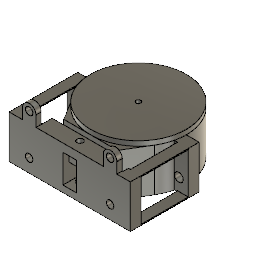
dropgen_assembly (Autodesk Fusion 360 archive; units mm, degrees)
design "drop_gen_reservoir"
Autodesk Fusion 360 part; units mm, degrees
sketch "Sketch1" plane through (0, 0, 0) normal (0, 1, 0) x (1, 0, 0) in component "reservoir assembly"
  line L0 (-25, 0) -> (25, 0)
  line L1 (25, 0) -> (25, 16)
  line L2 (25, 16) -> (-25, 16)
  line L3 (-25, 16) -> (-25, 0)
  line L4 (25, 0) -> (28.5, 0)
  line L5 (28.5, 0) -> (28.5, 19)
  line L6 (28.5, 19) -> (32, 19)
  line L7 (32, 19) -> (32, -5)
  line L8 (32, -5) -> (35.5, -5)
  line L9 (35.5, -5) -> (35.5, 27)
  line L10 (35.5, 27) -> (0, 27)
  line L11 (0, 0) -> (0, 27) construction
  line L12 (0, 16) -> (0, 27)
  line L13 (0, -8.5) -> (35.5, -8.5)
  line L14 (35.5, -8.5) -> (35.5, -5)
  line L15 (35.5, -5) -> (31.85, -5)
  line L16 (31.85, -5) -> (31.85, -3.5)
  line L17 (31.85, -3.5) -> (0, -3.5)
  line L18 (0, -3.5) -> (0, -8.5)
  line L19 (0, 16) -> (25, 8)
  line L20 (25, 0) -> (25, 8)
  dimension "d1" = 50
  dimension "d2" = 16
  dimension "d3" = 3.5
  dimension "d4" = 3.5
  dimension "d5" = 3.5
  dimension "d6" = 5
  dimension "d10" = 1.5
  dimension "d11" = 0.15
  dimension "d13" = 3.5
  dimension "d18" = 8
  dimension "d24" = 3
  dimension "d25" = 8
  constraint horizontal L0
  constraint vertical L1
  constraint horizontal L2
  constraint vertical L3
  constraint midpoint L11.start L0
  constraint perpendicular L1 L4
  constraint perpendicular L4 L5
  constraint perpendicular L5 L6
  constraint perpendicular L6 L7
  constraint perpendicular L7 L8
  constraint perpendicular L8 L9
  constraint perpendicular L9 L10
  constraint coincident L11.start origin
  constraint perpendicular L0 L11
  constraint midpoint L2 L12.start
  constraint parallel L2 L13
  constraint perpendicular L13 L14
  constraint perpendicular L14 L15
  constraint perpendicular L15 L16
  constraint perpendicular L16 L17
  constraint collinear L11 L18
  constraint coincident L1 L19.end
  measures "d1" distance of L0.start L0.end
  measures "d2" distance of L0.start L2.end
  measures "d3" distance of L0.end L4.end
  measures "d4" distance of L5.end L6.end
  measures "d5" distance of L7.end L8.end
  measures "d6" distance of L4 L8
  measures "d10" distance of L8 L17
  measures "d11" distance of L7 L16
  measures "d13" distance of L8.end L13.end
  measures "d18" distance of L6 L10
  measures "d24" vertical distance of L5.end L12.start
  measures "d25" distance of L0.end L19.end
revolve "Revolve1" add sketch "Sketch1" angle 360 about axis through (0, 0, 0) along (0, 0, -1) contours L1 L2 L4 L5 L6 L7 L8 L9 L10 L12 L15 L20 | L1 L2 L19 makes body 1 in component "reservoir assembly"
revolve "Revolve2" add sketch "Sketch1" angle 360 about axis through (0, 0, 0) along (0, 0, -1) separate body contours L8 L13 L14 L15 L16 L17 L18 makes body 2 in component "reservoir assembly"
sketch "Sketch2" plane through (0, 0, -27) normal (0, 0, -1) x (1, 0, 0) in component "reservoir assembly"
  circle A0 centre (0, 0) radius 32 construction
  circle A1 centre (0, 0) radius 28.5 construction
  circle A2 centre (0, 0) radius 3.925
  line L0 (-32, 0) -> (-28.5, 0) construction
  circle A3 centre (-30.25, 0) radius 3.925
  circle A4 centre (-30.25, 0) radius 1.75
  circle A5 centre (0, 0) radius 1.75
  circle A6 centre (0, 0) radius 25 construction
  circle A7 centre (0, 0) radius 25 construction
  dimension "d16" = 7.85
  dimension "d17" = 7.85
  dimension "d19" = 3.5
  dimension "d20" = 3.5
  constraint concentric A2 A6
  constraint coincident A0 L0.start
  constraint coincident A1 L0.end
  constraint horizontal L0
  constraint coincident A0.centre L0
  constraint midpoint L0 A3.centre
  constraint concentric A3 A4
  constraint concentric A0 A5
  measures "d16" diameter of A2
  measures "d17" diameter of A3
  measures "d19" diameter of A4
  measures "d20" diameter of A5
extrude "Extrude1" cut sketch "Sketch2" against normal through all contours A4 | A5 bodies 1 in component "reservoir assembly"
extrude "Extrude2" cut sketch "Sketch2" against normal blind 7 bodies 1 in component "reservoir assembly"
extrude "Extrude3" cut sketch "Sketch2" against normal up to surface (5 mm away) from surface at -30.5 contours A5 bodies 2 in component "reservoir assembly"
copy_body "Body->Comp1" bodies 1 removing the originals makes body 3 in component "reservoir"
copy_body "Body->Comp2" bodies 2 removing the originals makes body 4 in component "reservoir lid"
sketch "Sketch1 (2)" plane through (0, 0, -27) normal (0, 0, -1) x (1, 0, 0) in component "reservoir"
  circle A0 centre (-30.25, 0) radius 3.925
  circle A1 centre (0, 0) radius 3.925
  circle A2 centre (0, 0) radius 35.5
  line L0 (-35.5, 0) -> (-35.5, 35.5)
  line L1 (-35.5, 35.5) -> (35.5, 35.5)
  line L2 (35.5, 35.5) -> (35.5, 0)
  line L3 (37, 43) -> (45, 43)
  line L4 (45, 43) -> (45, 8)
  line L5 (45, 8) -> (37, 8)
  line L6 (37, 8) -> (37, 43)
  line L7 (35.5, 0) -> (45, 0)
  line L8 (45, 0) -> (45, 8)
  line L9 (45, 8) -> (35.5, 8)
  line L10 (35.5, 8) -> (35.5, 0)
  line L11 (-5, 35.5) -> (5, 35.5)
  line L12 (5, 35.5) -> (5, 47.5)
  line L13 (5, 47.5) -> (-5, 47.5)
  line L14 (-5, 47.5) -> (-5, 35.5)
  line L15 (45, 43) -> (45, 51)
  line L16 (45, 51) -> (0, 51)
  line L17 (37, 43) -> (35.5, 43)
  line L18 (35.5, 43) -> (35.5, 39)
  line L19 (35.5, 39) -> (0, 39)
  line L20 (0, 39) -> (0, 51) construction
  line L21 (-45, 43) -> (-45, 51)
  line L22 (-45, 51) -> (0, 51)
  line L23 (-35.5, 39) -> (0, 39)
  line L24 (-35.5, 43) -> (-35.5, 39)
  line L25 (-37, 43) -> (-45, 43)
  line L26 (-37, 8) -> (-37, 43)
  line L27 (-37, 43) -> (-35.5, 43)
  line L28 (-45, 43) -> (-45, 8)
  line L29 (-35.5, 0) -> (-45, 0)
  line L30 (-45, 0) -> (-45, 8)
  line L31 (-45, 8) -> (-35.5, 8)
  circle A3 centre (0, 43.25) radius 2.25
  line L32 (-5, 43.25) -> (5, 43.25) construction
  line L33 (4.5, 35.5) -> (4.5, 47)
  line L34 (4.5, 47) -> (-4.5, 47)
  line L35 (-4.5, 47) -> (-4.5, 35.5)
  line L36 (5, 47.5) -> (5, 51)
  line L37 (-5, 47.5) -> (-5, 51)
  line L38 (-20, 35.5) -> (-30.3629, 18.3941)
  line L39 (20, 35.5) -> (30.3629, 18.3941)
  line L40 (35.5, 8) -> (34.5868, 8)
  line L41 (-35.5, 8) -> (-34.5868, 8)
  dimension "d34" = 8
  dimension "d35" = 35
  dimension "d36" = 10
  dimension "d37" = 12
  dimension "d38" = 1.5
  dimension "d39" = 8
  dimension "d40" = 3.5
  dimension "d41" = 8
  dimension "d42" = 4.5
  dimension "d56" = 0.5
  dimension "d57" = 0.5
  dimension "d77" = 20
  constraint coincident A2 L0.start
  constraint tangent A2 L0
  constraint perpendicular L0 L1
  constraint coincident A2 L2.end
  constraint tangent A2 L2
  constraint perpendicular L1 L2
  constraint horizontal L1
  constraint tangent A2 L1
  constraint horizontal L3
  constraint vertical L4
  constraint horizontal L5
  constraint vertical L6
  constraint horizontal L7
  constraint vertical L8
  constraint horizontal L9
  constraint vertical L10
  constraint horizontal L11
  constraint vertical L12
  constraint horizontal L13
  constraint vertical L14
  constraint coincident L1 L11.start
  constraint midpoint L1 L11
  constraint perpendicular L3 L15
  constraint perpendicular L15 L16
  constraint perpendicular L6 L17
  constraint perpendicular L3 L18
  constraint perpendicular L12 L19
  constraint coincident A1.centre L20
  constraint vertical L20
  constraint collinear L2 L18
  constraint symmetric L2.end L20 L0.start
  constraint symmetric L3.start L20 L25.start
  constraint symmetric L3.end L20 L21.start
  constraint symmetric L4.end L20 L28.end
  constraint symmetric L5.end L20 L26.start
  constraint symmetric L7.end L20 L29.end
  constraint symmetric L9.end L20 L31.end
  constraint symmetric L15.end L20 L21.end
  constraint symmetric L16.end L20 L22.end
  constraint symmetric L17.end L20 L24.start
  constraint symmetric L18.end L20 L23.start
  constraint symmetric L19.end L20 L23.end
  constraint coincident L20 A3.centre
  constraint coincident L14 L32.start
  constraint coincident L12 L32.end
  constraint perpendicular L12 L32
  constraint coincident A3.centre L32
  constraint coincident L1 L33.start
  constraint perpendicular L1 L33
  constraint perpendicular L20 L34
  constraint coincident L11 L35.end
  constraint perpendicular L11 L35
  constraint symmetric L20 L33 L35
  constraint coincident L16 L36.end
  constraint perpendicular L16 L36
  constraint coincident L22 L37.end
  constraint perpendicular L22 L37
  constraint coincident L1 L38.start
  constraint coincident A2 L38.end
  constraint tangent A2 L38
  constraint symmetric L20 L38.start L39.start
  constraint symmetric L20 L38.end L39.end
  constraint coincident A2 L40.end
  constraint perpendicular L10 L40
  constraint coincident A2 L41.end
  constraint perpendicular L0 L41
  measures "d34" distance of L4.end L5.end
  measures "d35" distance of L3.start L5.end
  measures "d36" distance of L12.end L13.end
  measures "d37" distance of L11.start L13.end
  measures "d38" distance of L2 L6
  measures "d39" distance of L5 L7
  measures "d40" distance of L1 L19
  measures "d41" distance of L3.end L15.end
  measures "d42" diameter of A3
  measures "d56" distance of L14 L35
  measures "d57" distance of L13 L34
  measures "d77" horizontal distance of L19.end L38.start
extrude "Extrude1'" add sketch "Sketch1 (2)" against normal up to surface (32 mm away) contours A2 L2 L10 L40 | L2 L5 L7 L8 L9 L10 | A2 L0 L41 | L0 L29 L30 L31 | A2 L1 L11 L39 | A2 L1 L11 L38 | L3 L12 L15 L16 L17 L18 L19 L36 | L14 L21 L22 L23 L24 L25 L27 L37 | L13 L16 L22 L36 L37 bodies 3 makes body 5 at (15, -51, -16.3333) in component "reservoir"
extrude "Extrude2'" add sketch "Sketch1 (2)" against normal blind 0.8 contours L3 L4 L5 L6 L9 | L25 L26 L28 L31 bodies 3 5 in component "reservoir"
extrude "Extrude3'" add sketch "Sketch1 (2)" along normal blind 0.8 from surface at -32 contours L3 L4 L5 L6 L9 | L25 L26 L28 L31 bodies 3 in component "reservoir"
extrude "Extrude4" add sketch "Sketch1 (2)" along normal blind 6 from surface at -32 contours L19 L23 L33 L34 L35 | L12 L13 L14 L19 L23 L33 L34 L35 bodies 3 in component "reservoir"
extrude "Extrude5" add sketch "Sketch1 (2)" along normal blind 5 from surface at -23 contours L1 L11 L19 L23 L33 L35 | L19 L23 L33 L34 L35 | A3 bodies 3 in component "reservoir"
extrude "Extrude6" add sketch "Sketch1 (2)" along normal blind 1.5 from surface at -18 contours A3 bodies 3 in component "reservoir"
extrude "Extrude7" add sketch "Sketch1 (2)" against normal blind 5 contours L19 L23 L33 L34 L35 | L12 L13 L14 L19 L23 L33 L34 L35 bodies 3 in component "reservoir"
extrude "Extrude8" add sketch "Sketch1 (2)" against normal up to surface (6.5 mm away) contours A3 bodies 3 in component "reservoir"
extrude "Extrude9" cut sketch "Sketch1 (2)" against normal up to surface (21 mm away) from surface at -5 contours L13 L16 L22 L36 L37 bodies 3 in component "reservoir"
sketch "Sketch2 (2)" plane through (0, -51, 0) normal (0, -1, 0) x (1, 0, 0) in component "reservoir"
  line L0 (35.5, 5) -> (45, 5) construction
  line L1 (45, 5) -> (45, -27)
  line L2 (45, -27) -> (35.5, -27) construction
  line L3 (45, 5) -> (-45, 5) construction
  line L4 (0, 5) -> (0, -27) construction
  line L5 (0, -27) -> (35.5, -27) construction
  circle A0 centre (30, 13) radius 2.75
  circle A1 centre (30, -17) radius 2.75
  line L6 (45, 5) -> (25, 5)
  line L7 (25, 5) -> (25, 18)
  line L8 (25, 18) -> (45, 18)
  line L9 (45, 18) -> (45, 5)
  circle A2 centre (30, 13) radius 5
  circle A3 centre (30, -17) radius 5
  line L10 (35, 13) -> (35, 18)
  line L11 (30, 8) -> (25, 8)
  line L12 (35.5, -27) -> (35.5, 5)
  line L13 (30, -12) -> (45, -12)
  line L14 (30, -22) -> (45, -22)
  line L15 (25, 5) -> (25, -17)
  line L16 (35, 13) -> (35, -17)
  dimension "d68" = 5.5
  dimension "d69" = 30
  dimension "d70" = 5.5
  dimension "d71" = 30
  dimension "d72" = 8
  dimension "d73" = 5
  dimension "d74" = 20
  dimension "d75" = 10
  dimension "d76" = 10
  constraint midpoint L3 L4.start
  constraint perpendicular L3 L4
  constraint coincident L2.end L5.end
  constraint horizontal L5
  constraint vertical A0.centre A1.centre
  constraint horizontal L6
  constraint vertical L7
  constraint horizontal L8
  constraint vertical L9
  constraint coincident L0.end L1.start
  constraint concentric A0 A2
  constraint concentric A1 A3
  constraint coincident A2 L10.start
  constraint coincident A2 L11.start
  constraint coincident L7 L11.end
  constraint perpendicular L7 L11
  constraint coincident L8 L10.end
  constraint tangent A2 L10
  constraint perpendicular L8 L10
  constraint tangent A2 L11
  constraint coincident A3 L13.start
  constraint coincident L1 L13.end
  constraint perpendicular L1 L13
  constraint coincident A3 L14.start
  constraint coincident L1 L14.end
  constraint perpendicular L1 L14
  constraint tangent A3 L13
  constraint tangent A3 L14
  constraint coincident A3 L15.end
  constraint tangent A3 L15
  constraint coincident A3 L16.end
  constraint tangent A3 L16
  measures "d68" diameter of A0
  measures "d69" distance of L4 A0.centre
  measures "d70" diameter of A1
  measures "d71" distance of A0.centre A1.centre
  measures "d72" distance of L3 A0.centre
  measures "d73" distance of A0.centre L8
  measures "d74" distance of L7.end L8.end
  measures "d75" diameter of A2
  measures "d76" diameter of A3
extrude "Extrude10" add sketch "Sketch2 (2)" against normal blind 4 contours L6 L7 A2 L11 L16 | L8 A2 L10 | A2 | L7 L8 A2 | L7 A2 L11 bodies 3 in component "reservoir"
extrude "Extrude11" add sketch "Sketch2 (2)" against normal up to surface (4 mm away) from surface at -4 contours L6 L8 L9 L10 L16 | L6 L7 A2 L11 L16 bodies 3 in component "reservoir"
extrude "Extrude12" cut sketch "Sketch2 (2)" against normal up to surface (12 mm away) contours A1 bodies 3 in component "reservoir"
extrude "Extrude13" cut sketch "Sketch2 (2)" against normal up to surface (8 mm away) from surface at -4 contours L6 L8 L9 L10 L16 | L6 L12 L13 L16 | A3 L12 L13 L14 L16 | L6 A3 L13 L15 L16 | L6 L7 A2 L11 L16 | A3 L13 L16 | A3 bodies 3 in component "reservoir"
sketch "Sketch3" plane through (0, 0, 0) normal (0, 1, 0) x (-1, 0, 0) in component "reservoir"
  circle A0 centre (-30, -17) radius 2.75
  line L0 (-35.5, 5) -> (-45, 5)
  line L1 (-45, 5) -> (-45, -27)
  line L2 (-45, -27) -> (-35.5, -27)
  line L3 (-35.5, -27) -> (-35.5, 5)
  line L4 (-30, -17) -> (-45, -17) construction
  circle A1 centre (-38, -17) radius 2.5
  dimension "d93" = 5
  constraint coincident A0.centre L4.start
  constraint coincident L1 L4.end
  constraint perpendicular L1 L4
  constraint coincident L4 A1.centre
  constraint tangent L3 A1
  measures "d93" diameter of A1
extrude "Extrude14" cut sketch "Sketch3" against normal up to surface (8 mm away) draft 5 contours A1 bodies 3 in component "reservoir"
mirror "Mirror1" about plane through (0, 0, 0) normal (1, 0, 0) of "Extrude10", "Extrude11", "Extrude12", "Extrude13", "Extrude14" in component "reservoir"
fillet "Fillet1" radius 5 4 edges at (35, -49, 18) (25, -49, 18) (-25, -49, 18) (-35, -49, 18) on bodies 3 in component "reservoir"
component "reservoir assembly" placed x (1, 0, 0) y (0, 1, 0) z (0, 0, 1) at (0, 0, 0)
component "reservoir" placed x (1, 0, 0) y (0, 1, 0) z (0, 0, 1) at (0, 0, 0) in component "reservoir assembly"
component "reservoir lid" placed x (1, 0, 0) y (0, 1, 0) z (0, 0, 1) at (0, 0, 0) in component "reservoir assembly"
equation "d3 = wall_thickness"
equation "d4 = wall_thickness"
equation "d5 = wall_thickness"
equation "wall_thickness = 3.5 mm"
equation "d11 = toll"
equation "toll = 0.15 mm"
equation "d13 = wall_thickness"
equation "d19 = wall_thickness"
equation "d20 = wall_thickness"
equation "flex_width = 8 mm"
equation "flex_len = 35 mm"
equation "flex_thickness = 0.8 mm"
equation "d34 = flex_width"
equation "d35 = flex_len"
equation "d41 = d39"
equation "d45 = -flex_thickness"
equation "d48 = flex_thickness"
equation "d57 = d56"
equation "d70 = d68"

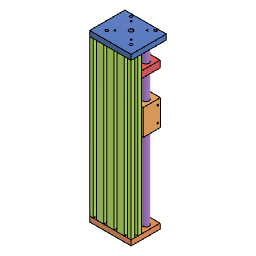
design "Linear actuator"
Autodesk Fusion 360 part; units mm, degrees
sketch "Sketch1" plane through (0, 0, 0) normal (0, 0, 1) x (1, 0, 0) in component "fixed components"
  line L0 (-40, 56) -> (40, 56)
  line L1 (40, 56) -> (40, 0)
  line L2 (40, 0) -> (-40, 0)
  line L3 (-40, 0) -> (-40, 56)
  circle A0 centre (0, 40) radius 6.5
  line L4 (0, 56) -> (0, 0) construction
  dimension "d1" = 80
  dimension "d2" = 56
  dimension "d3" = 13
  dimension "d4" = 40
  constraint horizontal L0
  constraint vertical L1
  constraint horizontal L2
  constraint vertical L3
  constraint midpoint L4.end L2
  constraint midpoint L0 L4.start
  constraint coincident L4.end origin
  constraint coincident A0.centre L4
  measures "d1" distance of L0.start L0.end
  measures "d2" distance of L0.start L2.end
  measures "d3" diameter of A0
  measures "d4" distance of L2 A0.centre
extrude "Extrude1" add sketch "Sketch1" along normal blind 10 makes body 1 in component "fixed components"
sketch "Sketch2" plane through (0, 0, 10) normal (0, 0, 1) x (-1, 0, 0) in component "fixed components"
  circle A0 centre (0, -40) radius 6.5
  line L0 (40, 0) -> (-40, 0)
  line L1 (-40, 0) -> (-40, -56)
  line L2 (-40, -56) -> (40, -56)
  line L3 (40, -56) -> (40, 0)
  line L4 (40, 0) -> (-40, 0)
  line L5 (-40, 0) -> (-40, -20)
  line L6 (-40, -20) -> (40, -20)
  line L7 (40, -20) -> (40, 0)
  line L8 (40, -13) -> (34, -13)
  line L9 (34, -13) -> (34, -7)
  line L10 (34, -7) -> (40, -7)
  line L11 (40, -7) -> (40, -13)
  line L12 (40, -10) -> (-40, -10) construction
  line L13 (33, -20) -> (27, -20)
  line L14 (27, -20) -> (27, -14)
  line L15 (27, -14) -> (33, -14)
  line L16 (33, -14) -> (33, -20)
  line L17 (13, -20) -> (7, -20)
  line L18 (7, -20) -> (7, -14)
  line L19 (7, -14) -> (13, -14)
  line L20 (13, -14) -> (13, -20)
  line L21 (30, -20) -> (30, -14) construction
  line L22 (10, -20) -> (10, -14) construction
  line L23 (33, -6) -> (33, 0)
  line L24 (33, 0) -> (27, 0)
  line L25 (27, -6) -> (33, -6)
  line L26 (27, 0) -> (27, -6)
  line L27 (7, 0) -> (7, -6)
  line L28 (7, -6) -> (13, -6)
  line L29 (13, 0) -> (7, 0)
  line L30 (13, -6) -> (13, 0)
  line L31 (0, -56) -> (0, 0) construction
  line L32 (-40, -13) -> (-34, -13)
  line L33 (-34, -13) -> (-34, -7)
  line L34 (-40, -7) -> (-40, -13)
  line L35 (-34, -7) -> (-40, -7)
  line L36 (-33, 0) -> (-27, 0)
  line L37 (-27, 0) -> (-27, -6)
  line L38 (-33, -6) -> (-33, 0)
  line L39 (-27, -6) -> (-33, -6)
  line L40 (-33, -20) -> (-27, -20)
  line L41 (-27, -20) -> (-27, -14)
  line L42 (-33, -14) -> (-33, -20)
  line L43 (-27, -14) -> (-33, -14)
  line L44 (-13, -20) -> (-7, -20)
  line L45 (-7, -20) -> (-7, -14)
  line L46 (-13, -14) -> (-13, -20)
  line L47 (-7, -14) -> (-13, -14)
  line L48 (-13, 0) -> (-7, 0)
  line L49 (-7, 0) -> (-7, -6)
  line L50 (-13, -6) -> (-13, 0)
  line L51 (-7, -6) -> (-13, -6)
  circle A1 centre (-28.5, -40) radius 6
  circle A2 centre (28.5, -40) radius 6
  dimension "d7" = 20
  dimension "d8" = 6
  dimension "d9" = 6
  dimension "d10" = 6
  dimension "d11" = 6
  dimension "d12" = 10
  dimension "d13" = 20
  dimension "d27" = 12
  dimension "d28" = 57
  constraint horizontal L4
  constraint vertical L5
  constraint horizontal L6
  constraint vertical L7
  constraint coincident L1 L5.end
  constraint coincident L0.start L3.end
  constraint horizontal L8
  constraint vertical L9
  constraint horizontal L10
  constraint vertical L11
  constraint coincident L3 L8.start
  constraint midpoint L11 L12.start
  constraint midpoint L5 L12.end
  constraint horizontal L12
  constraint horizontal L13
  constraint vertical L14
  constraint horizontal L15
  constraint vertical L16
  constraint coincident L6 L13.start
  constraint horizontal L17
  constraint vertical L18
  constraint horizontal L19
  constraint vertical L20
  constraint coincident L6 L17.start
  constraint equal L14 L20
  constraint equal L15 L19
  constraint midpoint L13 L21.start
  constraint midpoint L15 L21.end
  constraint midpoint L17 L22.start
  constraint midpoint L19 L22.end
  constraint symmetric L12 L13.start L23.end
  constraint symmetric L12 L13.end L24.end
  constraint symmetric L12 L14.end L25.start
  constraint symmetric L12 L15.end L23.start
  constraint symmetric L12 L17.start L29.start
  constraint symmetric L12 L17.end L27.start
  constraint symmetric L12 L18.end L27.end
  constraint symmetric L12 L19.end L28.end
  constraint symmetric L8.start L31 L32.start
  constraint symmetric L8.end L31 L32.end
  constraint symmetric L9.end L31 L33.end
  constraint symmetric L10.end L31 L34.start
  constraint symmetric L13.start L31 L40.start
  constraint symmetric L13.end L31 L40.end
  constraint symmetric L14.end L31 L41.end
  constraint symmetric L15.end L31 L42.start
  constraint symmetric L17.start L31 L44.start
  constraint symmetric L17.end L31 L44.end
  constraint symmetric L18.end L31 L45.end
  constraint symmetric L19.end L31 L46.start
  constraint symmetric L23.start L31 L38.start
  constraint symmetric L23.end L31 L36.start
  constraint symmetric L24.end L31 L36.end
  constraint symmetric L25.start L31 L37.end
  constraint symmetric L27.start L31 L48.end
  constraint symmetric L27.end L31 L49.end
  constraint symmetric L28.end L31 L50.start
  constraint symmetric L29.start L31 L48.start
  constraint symmetric L31 A1 A2
  constraint horizontal A0.centre A1.centre
  measures "d7" distance of L4 L6
  measures "d8" distance of L8.start L8.end
  measures "d9" distance of L8.start L10.end
  measures "d10" distance of L13.start L13.end
  measures "d11" distance of L13.start L15.end
  measures "d12" distance of L7 L21
  measures "d13" distance of L21 L22
  measures "d27" diameter of A1
  measures "d28" distance of A1.centre A2.centre
extrude "Extrude1'" add sketch "Sketch2" along normal blind 300 separate body contours L0 L1 L3 L4 L5 L6 L7 L8 L9 L10 L14 L15 L16 L18 L19 L20 L23 L25 L26 L27 L28 L30 L32 L33 L35 L37 L38 L39 L41 L42 L43 L45 L46 L47 L49 L50 L51 makes body 2 in component "Component"
copy_body "Body->Comp1" bodies 1 removing the originals makes body 3 in component "Component'"
sketch "Sketch3" plane through (0, 0, 310) normal (0, 0, 1) x (-1, 0, 0) in component "fixed components"
  circle A0 centre (0, -40) radius 6.5 construction
  line L0 (40, 0) -> (-40, 0)
  line L1 (-40, 0) -> (-40, -56)
  line L2 (-40, -56) -> (40, -56) construction
  line L3 (40, -56) -> (40, 0)
  line L4 (40, 0) -> (-40, 0)
  line L5 (-40, 0) -> (-40, -68)
  line L6 (-40, -68) -> (40, -68)
  line L7 (40, -68) -> (40, 0)
  line L8 (0, -40) -> (-40, 0) construction
  line L9 (0, -40) -> (0, 0) construction
  circle A1 centre (-15.5, -24.5) radius 1.5
  circle A2 centre (-23.5, -16.5) radius 2.5
  circle A3 centre (-23.5, -63.5) radius 2.5
  circle A4 centre (23.5, -63.5) radius 2.5
  circle A5 centre (23.5, -16.5) radius 2.5
  circle A6 centre (-15.5, -55.5) radius 1.5
  circle A7 centre (15.5, -55.5) radius 1.5
  circle A8 centre (15.5, -24.5) radius 1.5
  circle A9 centre (0, -40) radius 4
  dimension "d16" = 68
  dimension "d17" = 3
  dimension "d18" = 5
  dimension "d19" = 15.5
  dimension "d20" = 23.5
  dimension "d22" = 360
  dimension "d23" = 8
  constraint horizontal L4
  constraint vertical L5
  constraint horizontal L6
  constraint vertical L7
  constraint coincident L0.start L3.end
  constraint coincident L1.end L5
  constraint coincident A0.centre L8.start
  constraint coincident L0.end L1.start
  constraint coincident L9.end origin
  constraint coincident L8 A1.centre
  constraint coincident L8 A2.centre
  measures "d16" distance of L0.start L6.end
  measures "d17" diameter of A1
  measures "d18" diameter of A2
  measures "d19" distance of L9 A1.centre
  measures "d20" distance of L9 A2.centre
  measures "d23" diameter of A9
extrude "Extrude1''" add sketch "Sketch3" along normal blind 10 separate body makes body 4 in component "Component''"
ref_plane "WorkPlane1" through (0, 34, 282.5) normal (0, 0, -1) x (1, 0, 0) in component "fixed components"
extrude "Extrude1'''" add sketch "Sketch2" against normal blind 13 from surface at 272.5 separate body contours L1 L2 L3 L6 L13 L17 L40 L44 makes body 5 in component "Component'''"
extrude "Extrude1''''" add sketch "Sketch2" along normal up to surface (300 mm away) separate body contours A1 | A2 makes body 6 at (-34.4925, 40.2991, 210) makes body 7 at (22.5075, 40.2991, 210) in component "Component''''"
extrude "Extrude1'''''" add sketch "Sketch2" along normal up to surface (272.5 mm away) and the other way up to surface (10 mm away) separate body contours A0 makes body 8 in component "Component'''''"
ref_plane "WorkPlane1" through (0, 38, 219.5) normal (0, 0, -1) x (-1, 0, 0) in component "moving stage"
sketch "Sketch1 (2)" plane through (0, 0, 219.5) normal (0, 0, -1) x (-1, 0, 0) in component "moving stage"
  circle A0 centre (28.5, 40) radius 6
  circle A1 centre (-28.5, 40) radius 6
  circle A2 centre (0, 40) radius 6.5
  line L0 (-40, 20) -> (40, 20) construction
  line L1 (40, 20) -> (40, 56) construction
  line L2 (40, 56) -> (-40, 56) construction
  line L3 (-40, 56) -> (-40, 20) construction
  line L4 (-40, 56.5) -> (40, 56.5)
  line L5 (40, 56.5) -> (40, 23.5)
  line L6 (40, 23.5) -> (-40, 23.5)
  line L7 (-40, 23.5) -> (-40, 56.5)
  line L8 (40, 40) -> (-40, 40) construction
  dimension "d42" = 33
  constraint horizontal L4
  constraint vertical L5
  constraint horizontal L6
  constraint vertical L7
  constraint coincident L1 L5.end
  constraint midpoint L5 L8.start
  constraint midpoint L7 L8.end
  constraint coincident L2.end L7
  constraint coincident A2.centre L8
  measures "d42" distance of L4.end L5.end
extrude "Extrude1''''''" add sketch "Sketch1 (2)" along normal blind 50 separate body makes body 9 in component "moving stage"
sketch "Sketch2 (2)" plane through (0, 56.5, 0) normal (0, 1, 0) x (-1, 0, 0) in component "moving stage"
  line L0 (40, 219.5) -> (-40, 219.5)
  line L1 (-40, 219.5) -> (-40, 169.5)
  line L2 (-40, 169.5) -> (40, 169.5)
  line L3 (40, 169.5) -> (40, 219.5)
  line L4 (0, 219.5) -> (0, 169.5) construction
  line L5 (-40, 194.5) -> (40, 194.5) construction
  line L6 (-30, 209.5) -> (30, 209.5) construction
  line L7 (30, 209.5) -> (30, 179.5) construction
  line L8 (30, 179.5) -> (-30, 179.5) construction
  line L9 (-30, 179.5) -> (-30, 209.5) construction
  circle A0 centre (-30, 209.5) radius 2
  circle A1 centre (30, 209.5) radius 2
  circle A2 centre (30, 179.5) radius 2
  circle A3 centre (-30, 179.5) radius 2
  dimension "d45" = 30
  dimension "d46" = 60
  dimension "d47" = 4
  constraint midpoint L0 L4.start
  constraint midpoint L2 L4.end
  constraint midpoint L1 L5.start
  constraint midpoint L3 L5.end
  constraint horizontal L6
  constraint vertical L7
  constraint horizontal L8
  constraint vertical L9
  constraint symmetric L4 L7 L9
  constraint symmetric L5 L6 L8
  constraint coincident L6.start L9.end
  constraint coincident L6.end L7.start
  constraint coincident L7.end L8.start
  constraint coincident L8.end L9.start
  constraint equal A0 A1
  constraint equal A1 A2
  constraint equal A2 A3
  measures "d45" distance of L6.end L7.end
  measures "d46" distance of L7.end L8.end
  measures "d47" diameter of A0
extrude "Extrude2" cut sketch "Sketch2 (2)" against normal blind 8 contours A0 | A1 | A2 | A3 bodies 9 in component "moving stage"
sketch "Sketch3 (2)" plane through (40, 0, 0) normal (1, 0, 0) x (0, 1, 0) in component "moving stage"
  line L0 (56.5, 219.5) -> (23.5, 219.5)
  line L1 (23.5, 219.5) -> (23.5, 169.5)
  line L2 (23.5, 169.5) -> (56.5, 169.5)
  line L3 (56.5, 169.5) -> (56.5, 219.5)
  line L4 (56.5, 194.5) -> (23.5, 194.5) construction
  line L5 (51.5, 219.5) -> (51.5, 169.5) construction
  circle A0 centre (51.5, 209.5) radius 1.5
  circle A1 centre (51.5, 179.5) radius 1.5
  dimension "d50" = 5
  dimension "d51" = 3
  dimension "d52" = 15
  constraint midpoint L3 L4.start
  constraint midpoint L1 L4.end
  constraint coincident L0 L5.start
  constraint coincident L2 L5.end
  constraint perpendicular L2 L5
  constraint coincident L5 A0.centre
  constraint symmetric L4 A0 A1
  measures "d50" distance of L3 L5
  measures "d51" diameter of A0
  measures "d52" distance of L4 A0.centre
extrude "Extrude3" cut sketch "Sketch3 (2)" against normal blind 6 contours A0 | A1 bodies 9 in component "moving stage"
mirror "Mirror1" about plane through (0, 0, 0) normal (1, 0, 0) of "Extrude3" in component "moving stage"
component "fixed components" placed x (1, 0, 0) y (0, 1, 0) z (0, 0, 1) at (0, 0, 0)
component "moving stage" placed x (1, 0, 0) y (0, 1, 0) z (0, 0, 1) at (0, 0, 0)
component "Component" placed x (1, 0, 0) y (0, 1, 0) z (0, 0, 1) at (0, 0, 0) in component "fixed components"
component "Component'" placed x (1, 0, 0) y (0, 1, 0) z (0, 0, 1) at (0, 0, 0) in component "fixed components"
component "Component''" placed x (1, 0, 0) y (0, 1, 0) z (0, 0, 1) at (0, 0, 0) in component "fixed components"
component "Component'''" placed x (1, 0, 0) y (0, 1, 0) z (0, 0, 1) at (0, 0, 0) in component "fixed components"
component "Component''''" placed x (1, 0, 0) y (0, 1, 0) z (0, 0, 1) at (0, 0, 0) in component "fixed components"
component "Component'''''" placed x (1, 0, 0) y (0, 1, 0) z (0, 0, 1) at (0, 0, 0) in component "fixed components"
equation "d19 = ( 31 / 2 ) * 1 mm"
equation "d20 = ( 47 / 2 ) * 1 mm"
equation "d22 = 360.00 °"
equation "d40 = 0.00 °"
